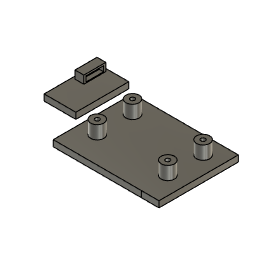
Golman v1 (Autodesk Fusion 360 design; units mm, degrees)
Autodesk Fusion 360 part; units mm, degrees
sketch "Sketch1" plane through (0, 0, 0) normal (0, 0, 1) x (1, 0, 0)
  line L0 (120.0463, 89.9645) -> (140.0463, 89.9645)
  line L1 (140.0463, -0.0355) -> (120.0463, -0.0355)
  line L2 (120.0463, -0.0355) -> (120.0463, 89.9645)
  line L3 (140.0463, 72.4645) -> (140.0463, 69.9645)
  circle A0 centre (140.0463, 69.9645) radius 2.5
  line L4 (140.0463, 69.9645) -> (140.0463, 67.4645)
  line L5 (140.0463, 32.4645) -> (140.0463, 29.9645)
  circle A1 centre (140.0463, 29.9645) radius 2.5
  line L6 (220.0463, 67.4645) -> (220.0463, 69.9645)
  line L7 (220.0463, 32.4645) -> (220.0463, 29.9645)
  circle A2 centre (220.0463, 69.9645) radius 2.5
  circle A3 centre (220.0463, 29.9645) radius 2.5
  line L8 (140.0463, 89.9645) -> (220, 89.9645)
  line L9 (220, 89.9645) -> (240, 89.9645)
  line L10 (240, 89.9645) -> (240, 40)
  line L11 (240, 40) -> (240, 0)
  line L12 (240, 0) -> (140, 0)
  line L13 (180.0463, 29.9645) -> (163.0463, 29.9645)
  line L14 (180.0463, 29.9645) -> (192.0463, 29.9645)
  line L15 (192.0463, 29.9645) -> (192.0463, 6.9645)
  line L16 (192.0463, 6.9645) -> (163.0463, 6.9645)
  line L17 (163.0463, 6.9645) -> (163.0463, 29.9645)
  line L18 (140.0463, 72.4645) -> (140.0463, 67.4645)
  line L19 (140.0463, 32.4645) -> (140.0463, 27.4645)
  line L20 (140.0463, 0) -> (140.0463, -0.0355)
  dimension "d1" = 20
  dimension "d2" = 90
  dimension "d3" = 20
  dimension "d4" = 5
  dimension "d8" = 5
  dimension "d17" = 5
  dimension "d18" = 5
  dimension "d21" = 17
  dimension "d22" = 12
  dimension "d23" = 23
  dimension "d24" = 29
  constraint horizontal L0
  constraint vertical L18
  constraint horizontal L1
  constraint vertical L2
  constraint perpendicular L0 L3
  constraint coincident L3.end A0.centre
  constraint parallel L4 L18
  constraint parallel L5 L18
  constraint coincident L5.end A1.centre
  constraint perpendicular L8 L18
  constraint perpendicular L9 L18
  constraint perpendicular L9 L10
  constraint perpendicular L12 L18
  constraint perpendicular L14 L15
  constraint perpendicular L15 L16
  constraint coincident A1 L5.start
  constraint collinear L18 L19
  constraint coincident A1 L19.end
  constraint coincident L12 L20.start
  constraint collinear L19 L20
  constraint coincident A3 L7.start
  constraint coincident A2 L6.start
  constraint coincident A0 L4.end
  constraint coincident A0 L3.start
  measures "d1" distance of L0.start L0.end
  measures "d2" distance of L0.start L1.end
  measures "d3" distance of L0.end L3.end
  measures "d4" diameter of A0
  measures "d8" diameter of A1
  measures "d17" diameter of A2
  measures "d18" diameter of A3
  measures "d21" distance of L13.start L13.end
  measures "d22" distance of L13.start L14.end
  measures "d23" distance of L14.end L15.end
  measures "d24" distance of L15.end L16.end
extrude "Extrude1" add sketch "Sketch1" along normal blind 7 makes body 1
sketch "Sketch2" plane through (0, 0, 7) normal (0, 0, 1) x (-1, 0, 0)
  circle A0 centre (-220.0463, -69.9645) radius 2.5
  line L0 (-163.0463, -29.9645) -> (-192.0463, -29.9645)
  line L1 (-192.0463, -29.9645) -> (-192.0463, -6.9645)
  line L2 (-192.0463, -6.9645) -> (-163.0463, -6.9645)
  line L3 (-163.0463, -6.9645) -> (-163.0463, -29.9645)
  circle A1 centre (-220.0463, -29.9645) radius 2.5
  circle A2 centre (-140.0463, -29.9645) radius 2.5
  circle A3 centre (-140.0463, -69.9645) radius 2.5
  line L4 (-140.0463, 0) -> (-240, 0)
  line L5 (-240, 0) -> (-240, -89.9645)
  line L6 (-240, -89.9645) -> (-120.0463, -89.9645)
  line L7 (-120.0463, -89.9645) -> (-120.0463, 0.0355)
  line L8 (-120.0463, 0.0355) -> (-140.0463, 0.0355)
  line L9 (-140.0463, 0.0355) -> (-140.0463, 0)
  line L10 (-163.0463, -29.9645) -> (-192.0463, -29.9645)
  line L11 (-192.0463, -29.9645) -> (-192.0463, -6.9645)
  line L12 (-192.0463, -6.9645) -> (-163.0463, -6.9645)
  line L13 (-163.0463, -6.9645) -> (-163.0463, -29.9645)
  constraint horizontal L10
  constraint vertical L11
  constraint horizontal L12
  constraint vertical L13
  constraint coincident L1.end L2.start
  constraint coincident L0.start L3.end
extrude "Extrude2" add sketch "Sketch2" against normal blind 4 contours L0 L1 L2 L3 L10 L11 L12 L13 bodies 1
extrude "Extrude3" add 1 faces at (172.7129, 14.6311, 3) along direction (0, 0, -1) blind 2 on bodies 1 bodies 1
extrude "Extrude4" cut 1 faces at (172.7129, 14.6311, 1) along direction (0, 0, 1) blind 50 on bodies 1 bodies 1
sketch "Sketch3" plane through (0, 0, 0) normal (0, 0, -1) x (1, 0, 0)
  circle A0 centre (220.0463, -69.9645) radius 2.5
  line L0 (192.0463, -29.9645) -> (163.0463, -29.9645)
  line L1 (163.0463, -29.9645) -> (163.0463, -6.9645)
  line L2 (163.0463, -6.9645) -> (192.0463, -6.9645)
  line L3 (192.0463, -6.9645) -> (192.0463, -29.9645)
  circle A1 centre (220.0463, -29.9645) radius 2.5
  circle A2 centre (140.0463, -29.9645) radius 2.5
  circle A3 centre (140.0463, -69.9645) radius 2.5
  line L4 (240, 0) -> (140.0463, 0)
  line L5 (140.0463, 0) -> (140.0463, 0.0355)
  line L6 (140.0463, 0.0355) -> (120.0463, 0.0355)
  line L7 (120.0463, 0.0355) -> (120.0463, -89.9645)
  line L8 (120.0463, -89.9645) -> (240, -89.9645)
  line L9 (240, -89.9645) -> (240, 0)
  line L10 (192.0463, -29.9645) -> (163.0463, -29.9645)
  line L11 (163.0463, -29.9645) -> (163.0463, -6.9645)
  line L12 (163.0463, -6.9645) -> (192.0463, -6.9645)
  line L13 (192.0463, -6.9645) -> (192.0463, -29.9645)
  constraint horizontal L10
  constraint vertical L11
  constraint horizontal L12
  constraint vertical L13
  constraint coincident L1.end L2.start
  constraint coincident L0.start L3.end
extrude "Extrude5" add sketch "Sketch3" against normal blind 4 contours L0 L1 L2 L3 L10 L11 L12 L13 bodies 1
sketch "Sketch4" plane through (0, 0, 0) normal (1, 0, 0) x (0, 1, 0)
sketch "Sketch5" plane through (0, 0, 7) normal (0, 0, 1) x (-1, 0, 0)
  line L0 (-163.0463, -6.9645) -> (-163.0463, -29.9645)
  line L1 (-163.0463, -29.9645) -> (-192.0463, -29.9645)
  line L2 (-192.0463, -29.9645) -> (-192.0463, -6.9645)
  line L3 (-192.0463, -6.9645) -> (-163.0463, -6.9645)
  circle A0 centre (-220.0463, -69.9645) radius 2.5
  circle A1 centre (-220.0463, -29.9645) radius 2.5
  circle A2 centre (-140.0463, -29.9645) radius 2.5
  circle A3 centre (-140.0463, -69.9645) radius 2.5
  line L4 (-140.0463, 0) -> (-240, 0)
  line L5 (-240, 0) -> (-240, -89.9645)
  line L6 (-240, -89.9645) -> (-120.0463, -89.9645)
  line L7 (-120.0463, -89.9645) -> (-120.0463, 0.0355)
  line L8 (-120.0463, 0.0355) -> (-140.0463, 0.0355)
  line L9 (-140.0463, 0.0355) -> (-140.0463, 0)
  line L10 (-50, -90) -> (-86, -90)
  line L11 (-86, -90) -> (-86, -30)
  line L12 (-86, -30) -> (-50, -30)
  line L13 (-50, -30) -> (-50, -90)
  dimension "d35" = 36
  dimension "d37" = 60
  constraint horizontal L10
  constraint vertical L11
  constraint horizontal L12
  constraint vertical L13
  measures "d35" distance of L10.start L10.end
  measures "d37" distance of L10.start L12.end
extrude "Extrude6" add sketch "Sketch5" along normal blind 7 separate body contours L10 L11 L12 L13 makes body 2
sketch "Sketch6" plane through (0, 0, 7) normal (0, 0, -1) x (1, 0, 0)
  line L0 (86, -30) -> (50, -30)
  line L1 (50, -30) -> (50, -90)
  line L2 (50, -90) -> (86, -90)
  line L3 (86, -90) -> (86, -30)
  line L4 (53.231, -87) -> (63, -87)
  line L5 (53.231, -87) -> (53, -87)
  line L6 (53, -87) -> (55, -87)
  line L7 (55, -87) -> (53, -87)
  line L8 (53, -87) -> (53, -78.5331)
  line L9 (53, -78.5331) -> (55, -78.5331)
  line L10 (55, -87) -> (58, -87)
  line L11 (58, -87) -> (63, -87)
  line L12 (63, -87) -> (58, -87)
  line L13 (58, -87) -> (58, -62)
  line L14 (58, -62) -> (63, -62)
  line L15 (63, -62) -> (63, -87)
  line L16 (58, -87) -> (53, -87)
  line L17 (53, -87) -> (53, -62)
  line L18 (53, -62) -> (58, -62)
  line L19 (58, -62) -> (58, -87)
  dimension "d42" = 2
  dimension "d43" = 3
  dimension "d44" = 5
  dimension "d45" = 25
  constraint perpendicular L3 L4
  constraint perpendicular L1 L5
  constraint horizontal L7
  constraint vertical L8
  constraint horizontal L9
  constraint parallel L4 L11
  constraint horizontal L12
  constraint vertical L13
  constraint horizontal L14
  constraint vertical L15
  constraint horizontal L16
  constraint vertical L17
  constraint horizontal L18
  constraint vertical L19
  measures "d42" distance of L6.end L5.end
  measures "d43" distance of L6.end L10.end
  measures "d44" distance of L10.end L4.end
  measures "d45" distance of L4.end L14.end
extrude "Extrude7" add sketch "Sketch6" along normal blind 7 contours L4 L5 L6 L7 L8 L10 L13 L16 L17 L18 L19 | L4 L11 L12 L13 L14 L15 L19 bodies 2
sketch "Sketch7" plane through (0, 0, 7) normal (0, 0, -1) x (1, 0, 0)
  line L0 (63, -62) -> (63, -87)
  line L1 (63, -87) -> (53, -87)
  line L2 (53, -87) -> (53, -62)
  line L3 (53, -62) -> (63, -62)
  line L4 (86, -30) -> (50, -30)
  line L5 (50, -30) -> (50, -90)
  line L6 (50, -90) -> (86, -90)
  line L7 (86, -90) -> (86, -30)
  line L8 (53, -87) -> (71, -87)
  line L9 (71, -87) -> (86, -87)
  line L10 (86, -87) -> (83, -87)
  line L11 (83, -87) -> (73, -87)
  line L12 (73, -87) -> (73, -62)
  line L13 (73, -62) -> (83, -62)
  line L14 (83, -62) -> (83, -87)
  dimension "d48" = 3
  dimension "d49" = 10
  dimension "d50" = 25
  constraint coincident L1.end L2.start
  constraint coincident L7 L9.end
  constraint perpendicular L7 L9
  constraint perpendicular L7 L10
  constraint horizontal L11
  constraint vertical L12
  constraint horizontal L13
  constraint vertical L14
  measures "d48" distance of L9.end L10.end
  measures "d49" distance of L10.end L11.end
  measures "d50" distance of L10.end L13.end
extrude "Extrude8" add sketch "Sketch7" along normal blind 7 contours L9 L11 L12 L13 L14 bodies 2
extrude "Extrude9" cut 1 faces at (59.6667, 75.8444, 0) along direction (0, 0, 1) blind 7 on bodies 2 bodies 2
sketch "Sketch8" plane through (73, 0, 0) normal (-1, 0, 0) x (0, -1, 0)
  line L0 (-62, 7) -> (-87, 7)
  line L1 (-87, 7) -> (-87, 0)
  line L2 (-87, 0) -> (-62, 0)
  line L3 (-62, 0) -> (-62, 7)
  line L4 (-87, 0) -> (-84.5, 0)
  line L5 (-84.5, 0) -> (-84.5, 7)
  line L6 (-62, 0) -> (-64.5, 0)
  line L7 (-64.5, 0) -> (-64.5, 7)
  line L8 (-74.5, 0) -> (-74.5, 2)
  line L9 (-74.5, 2) -> (-84.5, 2)
  line L10 (-64.5, 2) -> (-74.5, 2)
  line L11 (-64.5, 2) -> (-64.5, 9)
  dimension "d55" = 2.5
  dimension "d56" = 2.5
  dimension "d57" = 2
  dimension "d58" = 7
  constraint coincident L1.end L2.start
  constraint perpendicular L1 L4
  constraint coincident L0 L5.end
  constraint perpendicular L0 L5
  constraint coincident L2.end L3.start
  constraint perpendicular L3 L6
  constraint coincident L0 L7.end
  constraint perpendicular L0 L7
  constraint midpoint L2 L8.start
  constraint perpendicular L2 L8
  constraint coincident L5 L9.end
  constraint perpendicular L5 L9
  constraint coincident L7 L10.start
  constraint perpendicular L7 L10
  constraint perpendicular L10 L11
  measures "d55" distance of L1.end L4.end
  measures "d56" distance of L2.end L6.end
  measures "d57" distance of L8.start L8.end
  measures "d58" distance of L10.start L11.end
extrude "Extrude10" cut sketch "Sketch8" against normal blind 5 contours L0 L5 L7 L9 L10 L11 bodies 2
extrude "Extrude11" cut 1 faces at (69.6667, 40.6667, 7) along direction (0, 0, 1) blind 2 on bodies 2 bodies 2
extrude "Extrude12" add 1 faces at (62, 70, 14) along direction (0, 0, 1) blind 2 on bodies 2 bodies 2
sketch "Sketch9" plane through (78, 0, 0) normal (-1, 0, 0) x (0, -1, 0)
  line L0 (-84.5, 2) -> (-64.5, 2)
  line L1 (-64.5, 2) -> (-64.5, 9)
  line L2 (-64.5, 9) -> (-84.5, 9)
  line L3 (-84.5, 9) -> (-84.5, 2)
  line L4 (-69.5871, 9) -> (-69.5871, 7)
  line L5 (-69.5871, 7) -> (-64.5, 7)
  line L6 (-69.5871, 7) -> (-84.5, 7)
  constraint coincident L2 L4.start
  constraint perpendicular L2 L4
  constraint coincident L1 L5.end
  constraint perpendicular L1 L5
  constraint coincident L3 L6.end
  constraint perpendicular L3 L6
extrude "Extrude13" add sketch "Sketch9" along normal blind 5 contours L2 L3 L4 L6 | L1 L2 L4 L5 bodies 2
move_body "Move1" bodies 2 to x (-1, 0, 0) y (0, 1, 0) z (0, 0, -1) at (136, 10, 16)
sketch "Sketch10" plane through (0, 0, 0) normal (0, 0, -1) x (1, 0, 0)
  circle A0 centre (220.0463, -69.9645) radius 2.5
  circle A1 centre (220.0463, -29.9645) radius 2.5
  circle A2 centre (140.0463, -29.9645) radius 2.5
  circle A3 centre (140.0463, -69.9645) radius 2.5
  line L0 (240, 0) -> (140.0463, 0)
  line L1 (140.0463, 0) -> (140.0463, 0.0355)
  line L2 (140.0463, 0.0355) -> (120.0463, 0.0355)
  line L3 (120.0463, 0.0355) -> (120.0463, -89.9645)
  line L4 (120.0463, -89.9645) -> (240, -89.9645)
  line L5 (240, -89.9645) -> (240, 0)
  circle A4 centre (140.0463, -29.9645) radius 7.5
  circle A5 centre (140.0463, -69.9645) radius 7.5
  circle A6 centre (220.0463, -69.9645) radius 7.5
  circle A7 centre (220.0463, -29.9645) radius 7.5
  dimension "d67" = 15
  dimension "d68" = 15
  dimension "d69" = 15
  dimension "d70" = 15
  constraint concentric A2 A4
  constraint concentric A3 A5
  constraint concentric A0 A6
  constraint concentric A1 A7
  measures "d67" diameter of A4
  measures "d68" diameter of A5
  measures "d69" diameter of A6
  measures "d70" diameter of A7
extrude "Extrude14" add sketch "Sketch10" along normal blind 15 contours A4 | A5 | A6 | A7 bodies 1
sketch "Sketch11" plane through (0, 0, 0) normal (0, 0, -1) x (1, 0, 0)
  circle A0 centre (140.0463, -69.9645) radius 7.5
  circle A1 centre (220.0463, -69.9645) radius 7.5
  circle A2 centre (140.0463, -29.9645) radius 7.5
  circle A3 centre (220.0463, -29.9645) radius 7.5
  line L0 (240, 0) -> (140.0463, 0)
  line L1 (140.0463, 0) -> (140.0463, 0.0355)
  line L2 (140.0463, 0.0355) -> (120.0463, 0.0355)
  line L3 (120.0463, 0.0355) -> (120.0463, -89.9645)
  line L4 (120.0463, -89.9645) -> (240, -89.9645)
  line L5 (240, -89.9645) -> (240, 0)
move_body "Move2" bodies 1 to x (-1, 0, 0) y (0, 1, 0) z (0, 0, -1) at (340.3336, 0, 7.2628)
extrude "Extrude15" cut 1 faces at (59.6667, 87.8333, 9) along direction (0, 0, -1) blind 1 on bodies 2 bodies 2
